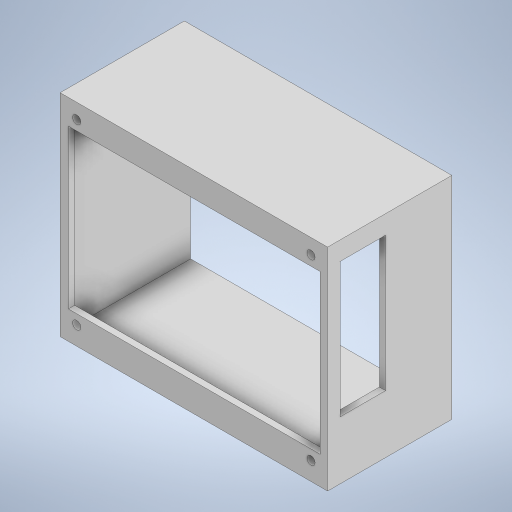
# Autodesk Inventor part: Behuizing
Saved by Autodesk Inventor 2023 (Build 270158000, 158)
## iProperties
Created: 2022-04-21
Part Number: Behuizing
Material: Generic
Document SubType Name: Modeling
Designer: Senne
Density: 1 g/cm^3
Appearance: Default
Author: Senne
## iProperties of the stored document Behuizing_3DPrint.ipt
Created: 2022-05-05
Part Number: Behuizing_3DPrint
Material: Generic
Document SubType Name: Modeling
Designer: Senne
Density: 1 g/cm^3
Appearance: Default
Author: Senne
Autodesk Inventor part; units mm, degrees
ref_plane "YZ Plane" through (0, 0, 0) normal (1, 0, 0) x (0, 1, 0)
ref_plane "XZ Plane" through (0, 0, 0) normal (0, 1, 0) x (-1, 0, 0)
ref_plane "XY Plane" through (0, 0, 0) normal (0, 0, 1) x (1, 0, 0)
sketch "Sketch1" plane through (0, 0, 0) normal (0, 1, 0) x (-1, 0, 0)
  line L0 (0, 0) -> (-125.15, 0)
  line L1 (-125.15, 0) -> (-125.15, -60)
  line L2 (-125.15, -60) -> (0, -60)
  line L3 (0, -60) -> (0, 0)
  dimension "d0" = 125.15
  dimension "d1" = 60
  constraints: 8 end point, 2 parallel, 1 horizontal, 1 perpendicular
  measures "d0" distance of L1.end L2.end
  measures "d1" distance of L0.end L1.end
extrude "Extrusion1" add sketch "Sketch1" along normal blind 100
sketch "Sketch2" plane through (0, 0, 0) normal (0, 0, 1) x (1, 0, 0)
  line L0 (2, 90) -> (123.51, 90)
  line L1 (123.51, 90) -> (123.51, 13.6)
  line L2 (123.51, 13.6) -> (2, 13.6)
  line L3 (2, 13.6) -> (2, 90)
  line L4 (0, 0) -> (125.15, 0) projected
  line L5 (0, 0) -> (0, 100) projected
  line L6 (0, 100) -> (125.15, 100) projected
  circle A0 centre (6.02, 94.765) radius 2
  circle A1 centre (6.02, 8.835) radius 2
  circle A2 centre (119.13, 94.765) radius 2
  circle A3 centre (119.13, 8.835) radius 2
  dimension "d4" = 76.4
  dimension "d5" = 121.51
  dimension "d7" = 2
  dimension "d15" = 10
  dimension "d16" = 4
  dimension "d17" = 4.765
  dimension "d18" = 4
  dimension "d19" = 85.93
  dimension "d21" = 4
  dimension "d22" = 113.11
  dimension "d23" = 6.02
  dimension "d24" = 4
  dimension "d25" = 4.765
  dimension "d26" = 113.11
  constraints: 8 end point, 4 centre point, 2 parallel, 1 horizontal, 1 perpendicular
  measures "d4" distance of L2.end L0.start
  measures "d5" distance of L1.end L2.end
  measures "d7" distance between parallel lines of L5 L3
  measures "d15" distance between parallel lines of L0 L6
  measures "d16" diameter of A0
  measures "d17" distance from line of L0 A0.centre
  measures "d18" diameter of A1
  measures "d19" distance of A0.centre A1.centre
  measures "d21" diameter of A2
  measures "d22" distance of A2.centre A0.centre
  measures "d23" distance from line of L5 A0.centre
  measures "d24" diameter of A3
  measures "d25" distance from line of L2 A3.centre
  measures "d26" distance of A3.centre A1.centre
extrude "Extrusion2" cut sketch "Sketch2" against normal blind 3
sketch "Sketch5" plane through (125.15, 0, 0) normal (1, 0, 0) x (0, 0, -1)
  line L0 (6, 93) -> (28, 93)
  line L1 (28, 93) -> (28, 28)
  line L2 (28, 28) -> (6, 28)
  line L3 (6, 28) -> (6, 93)
  line L4 (0, 100) -> (60, 100) projected
  line L5 (0, 0) -> (60, 0) projected
  line L6 (0, 0) -> (0, 100) projected
  point P0 (17, 93)
  point P1 (17, 28)
  dimension "d35" = 7
  dimension "d37" = 6
  dimension "d38" = 22
  dimension "d39" = 65
  constraints: 8 end point, 2 midpoint, 2 parallel, 1 horizontal, 1 perpendicular
  measures "d35" distance from line of L4 point (17, 93)
  measures "d37" distance between parallel lines of L6 L3
  measures "d38" distance of L1.end L2.end
  measures "d39" distance of L2.end L0.start
extrude "Extrusion4" cut sketch "Sketch5" against normal blind 10
sketch "Sketch7" plane through (125.15, 0, -60) normal (0, 0, -1) x (-1, 0, 0)
  line L0 (1, 99) -> (124.15, 99)
  line L1 (124.15, 99) -> (124.15, 4)
  line L2 (124.15, 4) -> (1, 4)
  line L3 (1, 4) -> (1, 99)
  line L4 (0, 100) -> (125.15, 100) projected
  line L5 (0, 0) -> (125.15, 0) projected
  line L6 (0, 0) -> (0, 100) projected
  line L7 (125.15, 0) -> (125.15, 100) projected
  dimension "d46" = 1
  dimension "d47" = 4
  dimension "d48" = 1
  dimension "d49" = 1
  constraints: 8 end point, 2 parallel, 1 horizontal, 1 perpendicular
  measures "d46" distance between parallel lines of L4 L0
  measures "d47" distance between parallel lines of L5 L2
  measures "d48" distance between parallel lines of L6 L3
  measures "d49" distance between parallel lines of L7 L1
extrude "Extrusion6" cut sketch "Sketch7" against normal blind 57 contours L0 L1 L2 L3
sketch "Sketch8" plane through (0, 100, 0) normal (0, 1, 0) x (1, 0, 0)
  line L0 (125.15, 0) -> (125.15, 60) projected
  line L1 (125.15, 60) -> (0, 60) projected
  line L2 (125.15, 0) -> (0, 0)
  line L3 (0, 0) -> (0, 60)
  line L4 (0, 60) -> (125.15, 60)
  line L5 (125.15, 60) -> (125.15, 0)
  point P0 (0, 0)
  constraints: 8 end point, 2 parallel, 1 horizontal, 1 perpendicular
extrude "Extrusion7" add sketch "Sketch8" along normal blind 2
sketch "Sketch9" plane through (125.15, 0, 0) normal (1, 0, 0) x (0, 0, -1)
  line L0 (0, 0) -> (60, 0) projected
  line L1 (0, 102) -> (60, 102)
  line L2 (60, 102) -> (60, 0)
  line L3 (60, 0) -> (0, 0)
  line L4 (0, 0) -> (0, 102)
  line L5 (6, 93) -> (28, 93) projected
  line L6 (28, 93) -> (28, 28) projected
  line L7 (6, 93) -> (28, 93)
  line L8 (28, 93) -> (28, 28)
  line L9 (28, 28) -> (6, 28)
  line L10 (6, 28) -> (6, 93)
  constraints: 16 end point, 4 parallel, 2 horizontal, 2 perpendicular
extrude "Extrusion8" add sketch "Sketch9" along normal blind 2
sketch "Sketch10" plane through (0, 0, -60) normal (-1, 0, 0) x (0, 0, 1)
  line L0 (0, 0) -> (0, 102) projected
  line L1 (60, 0) -> (60, 102) projected
  line L2 (0, 102) -> (60, 102)
  line L3 (60, 102) -> (60, 0)
  line L4 (60, 0) -> (0, 0)
  line L5 (0, 0) -> (0, 102)
  constraints: 8 end point, 2 parallel, 1 horizontal, 1 perpendicular
extrude "Extrusion9" add sketch "Sketch10" along normal blind 2
body "Solid1"
